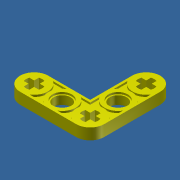
# Autodesk Inventor part: LEGO Brick 32017
Saved by Autodesk Inventor 2011 SP2 (Build 150553200, 553)
## iProperties
Company: Allseas Engineering BV
Created: 2011-11-29
Part Number: LEGO Brick 32017
Cost Center: 0 kg
Material: Steel
Document SubType Name: Modeling
Designer: BvH
Authority: 0 mm^3
Stock Number: =<Filenr>_<Document number>
Density: 7.85 g/cm^3
Act. Code: DW000
SaveDate: 2011-07-28
SaveTime: 18:32
FileName: Standard
TotalMass: 0 kg
TotalVolume: 0 mm^3
Subject: =<Title><TITLE 1_2> <TITLE 2_2>
Author: BvH
Autodesk Inventor part; units mm, degrees
ref_plane "YZ Plane" through (0, 0, 0) normal (1, 0, 0) x (0, 1, 0)
ref_plane "XZ Plane" through (0, 0, 0) normal (0, 1, 0) x (-1, 0, 0)
ref_plane "XY Plane" through (0, 0, 0) normal (0, 0, 1) x (1, 0, 0)
sketch "Sketch1" plane through (0, 0, 0) normal (0, 0, 1) x (1, 0, 0)
  line L0 (0, -9.7941) -> (0, 24.9657) construction
  line L1 (-24.9657, 0) -> (9.7941, 0) construction
  line L2 (-4, 4) -> (-4, 16)
  arc A0 (4, 16) -> (-4, 16) centre (0, 16) ccw
  line L3 (4, 16) -> (4, 0)
  arc A1 (0, -4) -> (4, 0) centre (0, 0) ccw
  line L4 (0, -4) -> (-16, -4)
  arc A2 (-16, 4) -> (-16, -4) centre (-16, 0) ccw
  line L5 (-16, 4) -> (-4, 4)
  dimension "d38" = 8
  dimension "d39" = 24
  constraints: 8 end point, 6 point on circle, 6 tangent, 4 point on line, 3 centre point, 2 horizontal, 2 vertical, 1 perpendicular
  measures "d38" distance between parallel lines of L3 L2
sketch "Sketch6" plane through (0, 0, 0) normal (0, 0, 1) x (1, 0, 0)
  circle A0 centre (-16, 0) radius 2.3
  circle A1 centre (0, 16) radius 2.3
  line L0 (-18.1564, 0.8) -> (-16.8, 0.8)
  line L1 (-16.8, 0.8) -> (-16.8, 2.1564)
  line L2 (-15.2, 2.1564) -> (-15.2, 0.8)
  line L3 (-15.2, 0.8) -> (-13.8436, 0.8)
  line L4 (-13.8436, -0.8) -> (-15.2, -0.8)
  line L5 (-15.2, -0.8) -> (-15.2, -2.1564)
  line L6 (-16.8, -2.1564) -> (-16.8, -0.8)
  line L7 (-16.8, -0.8) -> (-18.1564, -0.8)
  line L8 (-2.1564, 16.8) -> (-0.8, 16.8)
  line L9 (0.8, 16.8) -> (2.1564, 16.8)
  line L10 (0.8, 18.1564) -> (0.8, 16.8)
  line L11 (0.8, 15.2) -> (0.8, 13.8436)
  line L12 (-0.8, 18.1564) -> (-0.8, 16.8)
  line L13 (-0.8, 15.2) -> (-0.8, 13.8436)
  line L14 (2.1564, 15.2) -> (0.8, 15.2)
  line L15 (-0.8, 15.2) -> (-2.1564, 15.2)
  arc A2 (0, -4) -> (4, 0) centre (0, 0) ccw construction
  arc A3 (4, 16) -> (-4, 16) centre (0, 16) ccw construction
  arc A4 (-16, 4) -> (-16, -4) centre (-16, 0) ccw construction
  circle A5 centre (0, 0) radius 2.3
  line L16 (-2.1564, 0.8) -> (-0.8, 0.8)
  line L17 (-0.8, 0.8) -> (-0.8, 2.1564)
  line L18 (0.8, 2.1564) -> (0.8, 0.8)
  line L19 (0.8, 0.8) -> (2.1564, 0.8)
  line L20 (2.1564, -0.8) -> (0.8, -0.8)
  line L21 (0.8, -0.8) -> (0.8, -2.1564)
  line L22 (-0.8, -2.1564) -> (-0.8, -0.8)
  line L23 (-0.8, -0.8) -> (-2.1564, -0.8)
  circle A6 centre (0, 0) radius 2.75
  circle A7 centre (-16, 0) radius 2.75
  circle A8 centre (0, 16) radius 2.75
  dimension "d40" = 4.6
  dimension "d41" = 1.6
  dimension "d50" = 5.5
  constraints: 48 end point, 19 equal length, 12 horizontal, 12 vertical, 6 coincident, 4 collinear, 3 centre point, 2 equal radius, 30 other
  measures "d41" distance between parallel lines of L18 L17
  measures "d50" diameter of A6
sketch "Sketch8" plane through (0, 0, 0) normal (0, 0, 1) x (1, 0, 0)
  arc A0 (0, -4) -> (4, 0) centre (0, 0) ccw construction
  line L0 (0, -8.9941) -> (0, 20.1657) construction
  line L1 (-20.1657, 0) -> (8.9941, 0) construction
  circle A1 centre (0, 8) radius 2.4
  circle A2 centre (-8, 0) radius 2.4
  circle A3 centre (0, 8) radius 2.75
  circle A4 centre (-8, 0) radius 2.75
  line L2 (0, -4) -> (-16, -4) construction
  line L3 (4, 16) -> (4, 0) construction
  point P0 (4, 8)
  point P1 (-8, -4)
  dimension "d42" = 4.8
  dimension "d43" = 5.5
  constraints: 4 centre point, 2 coincident, 2 equal radius, 2 midpoint, 2 point on line, 1 horizontal alignment, 1 vertical alignment
  measures "d42" diameter of A1
  measures "d43" diameter of A3
extrude "Extrusion1" add sketch "Sketch1" along normal mid plane 3.2
extrude "Extrusion9" cut sketch "Sketch6" along normal through all both and the other way through all contours A0 L4 L5 L6 L7 L0 L1 L2 L3 | A1 L14 L11 L13 L15 L8 L12 L10 L9 | A5 L20 L21 L22 L23 L16 L17 L18 L19
extrude "Extrusion10" cut sketch "Sketch8" along normal through all both and the other way through all contours A1 | A2
sketch "Sketch3" plane through (0, 0, 1.6) normal (0, 0, 1) x (1, 0, 0)
  circle A0 centre (-8, 0) radius 2.75 projected
  circle A1 centre (0, 8) radius 2.75 projected
extrude "Extrusion4" cut sketch "Sketch3" against normal blind 0.5333
sketch "Sketch9" plane through (0, 0, -1.6) normal (0, 0, -1) x (-1, 0, 0)
  circle A0 centre (8, 0) radius 2.75 projected
  circle A1 centre (0, 8) radius 2.75 projected
extrude "Extrusion11" cut sketch "Sketch9" against normal blind 0.5333
sketch "Sketch4" plane through (0, 0, 1.6) normal (0, 0, 1) x (1, 0, 0)
  circle A0 centre (-16, 0) radius 2.3 construction
  circle A1 centre (0, 16) radius 2.3 construction
  arc A2 (-5.9892, -3.3333) -> (-5.9892, 3.3333) centre (-8, 0) ccw
  line L0 (-5.9892, 3.3333) -> (-2.0108, 3.3333)
  line L1 (-5.9892, -3.3333) -> (-2.0108, -3.3333)
  arc A3 (-2.0108, 3.3333) -> (-2.0108, -3.3333) centre (0, 0) ccw
  circle A4 centre (0, 0) radius 2.75 construction
  circle A5 centre (0, 16) radius 2.75 construction
  circle A6 centre (-16, 0) radius 2.75 construction
  line L2 (0, -9.5229) -> (0, 24.9205) construction
  line L3 (-25.4536, 0) -> (12.7217, 0) construction
  circle A7 centre (-8, 0) radius 2.75 construction
  circle A8 centre (0, 8) radius 2.75 construction
  arc A9 (-10.0108, 3.3333) -> (-10.0108, -3.3333) centre (-8, 0) ccw
  arc A10 (-13.9892, -3.3333) -> (-13.9892, 3.3333) centre (-16, 0) ccw
  line L4 (-10.0108, -3.3333) -> (-13.9892, -3.3333)
  line L5 (-10.0108, 3.3333) -> (-13.9892, 3.3333)
  arc A11 (3.3333, 2.0108) -> (-3.3333, 2.0108) centre (0, 0) ccw
  arc A12 (-3.3333, 5.9892) -> (3.3333, 5.9892) centre (0, 8) ccw
  line L6 (3.3333, 2.0108) -> (3.3333, 5.9892)
  line L7 (-3.3333, 2.0108) -> (-3.3333, 5.9892)
  line L8 (3.3333, 10.0108) -> (3.3333, 13.9892)
  line L9 (-3.3333, 10.0108) -> (-3.3333, 13.9892)
  arc A13 (-3.3333, 13.9892) -> (3.3333, 13.9892) centre (0, 16) ccw
  arc A14 (3.3333, 10.0108) -> (-3.3333, 10.0108) centre (0, 8) ccw
  dimension "d33" = 6.6667
  dimension "d51" = 1.1429
  dimension "d52" = 6.6667
  constraints: 16 end point, 16 point on circle, 8 centre point, 8 coincident, 7 equal radius, 4 collinear, 4 horizontal, 4 vertical, 2 parallel, 1 point on line
  measures "d33" distance between parallel lines of L1 L0
  measures "d51" radial gap between concentric circles of A3 A4
  measures "d52" distance between parallel lines of L7 L6
extrude "Extrusion5" cut sketch "Sketch4" against normal blind 0.5333
sketch "Sketch10" plane through (0, 0, -1.6) normal (0, 0, -1) x (-1, 0, 0)
  arc A0 (-3.3333, 13.9892) -> (3.3333, 13.9892) centre (0, 16) ccw projected
  line L0 (3.3333, 13.9892) -> (3.3333, 10.0108) projected
  arc A1 (3.3333, 10.0108) -> (-3.3333, 10.0108) centre (0, 8) ccw projected
  line L1 (-3.3333, 10.0108) -> (-3.3333, 13.9892) projected
  arc A2 (2.0108, -3.3333) -> (-3.3333, 2.0108) centre (0, 0) ccw projected
  line L2 (-3.3333, 2.0108) -> (-3.3333, 5.9892) projected
  arc A3 (-3.3333, 5.9892) -> (3.3333, 5.9892) centre (0, 8) ccw projected
  line L3 (3.3333, 5.9892) -> (3.3333, 3.3333) projected
  line L4 (3.3333, 3.3333) -> (5.9892, 3.3333) projected
  arc A4 (5.9892, 3.3333) -> (5.9892, -3.3333) centre (8, 0) ccw projected
  line L5 (5.9892, -3.3333) -> (2.0108, -3.3333) projected
  line L6 (10.0108, 3.3333) -> (13.9892, 3.3333) projected
  arc A5 (13.9892, 3.3333) -> (13.9892, -3.3333) centre (16, 0) ccw projected
  line L7 (13.9892, -3.3333) -> (10.0108, -3.3333) projected
  arc A6 (10.0108, -3.3333) -> (10.0108, 3.3333) centre (8, 0) ccw projected
extrude "Extrusion12" cut sketch "Sketch10" against normal blind 0.5333
equation "\"d38\" = width_standard"
equation "\"d2\" = 0.333333 * height_standard"
equation "\"d15\" = 0.0555556 * height_standard"
equation "\"d48\" = 0.0555556 * height_standard"
equation "\"d33\" = 0.833333 * width_standard"
equation "\"d52\" = 0.833333 * width_standard"
equation "\"d20\" = 0.0555556 * height_standard"
equation "\"d53\" = 0.0555556 * height_standard"
equation "\"width_standard\" = 8"
equation "\"height_standard\" = 9.6"
body "Solid1"
